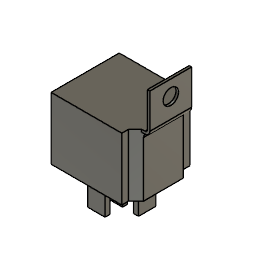
Base (Autodesk Fusion 360 archive; units mm, degrees)
design "Relay BB"
Autodesk Fusion 360 part; units mm, degrees
sketch "Sketch1" plane through (0, 0, 0) normal (0, 0, 1) x (1, 0, 0)
  line L0 (14.2, -13.7) -> (-14.2, -13.7)
  line L1 (-14.2, -13.7) -> (-14.2, 13.7)
  line L2 (-14.2, 13.7) -> (14.2, 13.7)
  line L3 (14.2, 13.7) -> (14.2, -13.7)
  line L4 (14.2, -13.7) -> (-14.2, 13.7) construction
  line L5 (-14.2, -13.7) -> (14.2, 13.7) construction
  dimension "d1" = 28.4
  dimension "d2" = 27.4
  constraint horizontal L0
  constraint perpendicular L0 L1
  constraint parallel L0 L2
  constraint parallel L1 L3
  constraint coincident L4 origin
  constraint coincident L5 origin
  measures "d1" distance of L1.end L2.end
  measures "d2" distance of L0.end L1.end
extrude "Extrude1" add sketch "Sketch1" along normal blind 25
sketch "Sketch2" plane through (14.2, 0, 0) normal (1, 0, 0) x (0, 1, 0)
  line L0 (-13.7, 0) -> (13.7, 0)
  line L1 (13.7, 0) -> (13.7, 25)
  line L2 (13.7, 25) -> (-13.7, 25)
  line L3 (-13.7, 25) -> (-13.7, 0)
  line L4 (0, 25) -> (8.4, 25)
  line L5 (8.4, 25) -> (8.4, 40)
  line L6 (8.4, 40) -> (0, 40)
  line L7 (0, 40) -> (0, 25)
  line L8 (0, 40) -> (-8.4, 40)
  line L9 (-8.4, 40) -> (-8.4, 25)
  line L10 (-8.4, 25) -> (0, 25)
  line L11 (0, 25) -> (0, 40)
  dimension "d5" = 8.4
  dimension "d6" = 15
  dimension "d7" = 8.4
  constraint horizontal L4
  constraint vertical L5
  constraint horizontal L6
  constraint vertical L7
  constraint midpoint L2 L4.start
  constraint horizontal L8
  constraint vertical L9
  constraint horizontal L10
  constraint vertical L11
  constraint coincident L2 L9.end
  measures "d5" distance of L4.start L4.end
  measures "d6" distance of L4.start L6.end
  measures "d7" distance of L6.end L8.end
extrude "Extrude2" add sketch "Sketch2" against normal blind 2 contours L2 L7 L8 L9 L10 L11 | L2 L4 L5 L6 L7 L11
sketch "Sketch3" plane through (14.2, 0, 0) normal (1, 0, 0) x (0, 1, 0)
  line L0 (-13.7, 0) -> (13.7, 0)
  line L1 (13.7, 0) -> (13.7, 25)
  line L2 (13.7, 25) -> (8.4, 25)
  line L3 (-8.4, 25) -> (-13.7, 25)
  line L4 (-13.7, 25) -> (-13.7, 0)
  line L5 (-8.4, 25) -> (8.4, 25)
  line L6 (0, 40) -> (0, 33.9)
  circle A0 centre (0, 33.9) radius 3.1
  line L7 (8.4, 25) -> (8.4, 40)
  line L8 (8.4, 40) -> (-8.4, 40)
  line L9 (-8.4, 40) -> (-8.4, 25)
  dimension "d10" = 6.1
  dimension "d11" = 6.2
  constraint coincident L3.start L5.start
  constraint coincident L2.end L5.end
  constraint coincident L6.end A0.centre
  measures "d10" distance of L6.start L6.end
  measures "d11" diameter of A0
extrude "Extrude3" cut sketch "Sketch3" against normal blind 30 contours A0
sketch "Sketch4" plane through (0, 0, 0) normal (0, 0, 1) x (1, 0, 0)
  line L0 (-3.2, -10) -> (3.8, -10)
  line L1 (3.8, -10) -> (3.8, -8)
  line L2 (3.8, -8) -> (-3.2, -8)
  line L3 (-3.2, -8) -> (-3.2, -10)
  line L4 (-10.2, -3) -> (-8.2, -3)
  line L5 (-8.2, -3) -> (-8.2, 4)
  line L6 (-8.2, 4) -> (-10.2, 4)
  line L7 (-10.2, 4) -> (-10.2, -3)
  line L8 (8.2, -3) -> (10.2, -3)
  line L9 (10.2, -3) -> (10.2, 4)
  line L10 (10.2, 4) -> (8.2, 4)
  line L11 (8.2, 4) -> (8.2, -3)
  line L12 (-3.2, 7.7) -> (3.8, 7.7)
  line L13 (3.8, 7.7) -> (3.8, 9.7)
  line L14 (3.8, 9.7) -> (-3.2, 9.7)
  line L15 (-3.2, 9.7) -> (-3.2, 7.7)
  line L16 (-3.2, -3) -> (3.8, -3)
  line L17 (3.8, -3) -> (3.8, -1)
  line L18 (3.8, -1) -> (-3.2, -1)
  line L19 (-3.2, -1) -> (-3.2, -3)
  line L20 (-14.2, 13.7) -> (14.2, 13.7)
  line L21 (14.2, 13.7) -> (14.2, -13.7)
  line L22 (14.2, -13.7) -> (-14.2, -13.7)
  line L23 (-14.2, -13.7) -> (-14.2, 13.7)
  dimension "d14" = 4
  dimension "d15" = 4
  dimension "d16" = 4
  dimension "d17" = 11
  dimension "d18" = 11
  dimension "d19" = 11
  constraint horizontal L0
  constraint vertical L1
  constraint horizontal L2
  constraint vertical L3
  constraint horizontal L4
  constraint vertical L5
  constraint horizontal L6
  constraint vertical L7
  constraint horizontal L8
  constraint vertical L9
  constraint horizontal L10
  constraint vertical L11
  constraint horizontal L12
  constraint vertical L13
  constraint horizontal L14
  constraint vertical L15
  constraint horizontal L16
  constraint vertical L17
  constraint horizontal L18
  constraint vertical L19
  measures "d14" distance of L9 L21
  measures "d15" distance of L7 L23
  measures "d16" distance of L14 L20
  measures "d17" distance of L15 L23
  measures "d18" distance of L3 L23
  measures "d19" distance of L19 L23
extrude "Extrude4" add sketch "Sketch4" against normal blind 11.3 contours L0 L1 L2 L3 | L4 L5 L6 L7 | L8 L9 L10 L11 | L12 L13 L14 L15 | L16 L17 L18 L19
extrude "Extrude5" add sketch "Sketch3" along normal blind 1 contours L5 L7 L8 L9
sketch "Sketch5" plane through (14.2, 0, 0) normal (1, 0, 0) x (0, 1, 0)
  line L0 (8.4, 25) -> (-8.4, 25)
  line L1 (-8.4, 25) -> (-13.7, 25)
  line L2 (-13.7, 25) -> (-13.7, 0)
  line L3 (-13.7, 0) -> (13.7, 0)
  line L4 (13.7, 0) -> (13.7, 25)
  line L5 (13.7, 25) -> (8.4, 25)
  line L6 (0, 25) -> (11, 25)
  line L7 (11, 25) -> (11, 0)
  line L8 (11, 0) -> (0, 0)
  line L9 (0, 0) -> (0, 25)
  line L10 (0, 25) -> (-11, 25)
  line L11 (-11, 25) -> (-11, 0)
  line L12 (-11, 0) -> (0, 0)
  line L13 (0, 0) -> (0, 25)
  dimension "d26" = 11
  constraint horizontal L6
  constraint vertical L7
  constraint horizontal L8
  constraint vertical L9
  constraint midpoint L0 L6.start
  constraint coincident L3 L7.end
  constraint horizontal L10
  constraint vertical L11
  constraint horizontal L12
  constraint vertical L13
  constraint coincident L3 L11.end
  measures "d26" distance of L6.start L6.end
extrude "Extrude7" add sketch "Sketch5" along normal blind 3 contours L0 L3 L5 L6 L7 L8 L9 L13 | L0 L1 L3 L9 L10 L11 L12 L13
chamfer "Chamfer1" distance 3 angle 45 2 edges at (17.2, -11, 12.5) (17.2, 11, 12.5)
extrude "Extrude8" add 1 faces at (15.2, 0.0772, 26.9362) along direction (1, 0, 0) blind 5
extrude "Extrude9" add 1 faces at (19.2, 2.6669, 25) along direction (0, 0, -1) blind 1
extrude "Extrude10" cut 1 faces at (12.2, -0.0772, 26.9362) along direction (1, 0, 0) blind 7
fillet "Fillet1" radius 2 1 edges at (20.2, 0, 24)
fillet "Fillet2" radius 1 1 edges at (19.2, 0, 25)
fillet "Fillet3" radius 2 1 edges at (17.2, 0, 24)
equation "d5 = ( 16.8 / 2 ) * 1 mm"
equation "d26 = ( 22 / 2 ) * 1 mm"

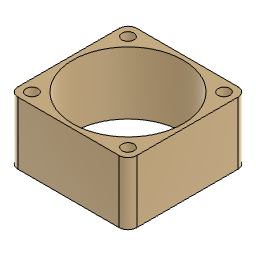
design "noctua_fan_40mm"
Autodesk Fusion 360 part; units mm, degrees
box "BoxPrimitive1" add length 40 width 40 height 21 placed x (0, -1, 0) y (1, 0, 0) z (0, 0, 1) at (40, 0, 0)
fillet "Fillet1" radius 3 4 edges at (40, -40, 10.5) (80, -40, 10.5) (80, 0, 10.5) (40, 0, 10.5)
sketch "Sketch2" plane through (0, 0, 21) normal (0, 0, 1) x (-1, 0, 0)
  arc A0 (-43, 0) -> (-40, 3) centre (-43, 3) ccw
  line L0 (-40, 3) -> (-40, 37)
  arc A1 (-40, 37) -> (-43, 40) centre (-43, 37) ccw
  line L1 (-43, 40) -> (-77, 40)
  arc A2 (-77, 40) -> (-80, 37) centre (-77, 37) ccw
  line L2 (-80, 37) -> (-80, 3)
  arc A3 (-80, 3) -> (-77, 0) centre (-77, 3) ccw
  line L3 (-77, 0) -> (-43, 0)
  circle A4 centre (-76.15, 36.15) radius 2
  circle A5 centre (-76.15, 3.85) radius 2
  circle A6 centre (-43.85, 36.15) radius 2
  circle A7 centre (-43.85, 3.85) radius 2
  line L4 (-40.8787, 0.8787) -> (-79.1213, 39.1213) construction
  line L5 (-40.8787, 39.1213) -> (-79.1213, 0.8787) construction
  circle A8 centre (-60, 20) radius 18.55
  dimension "d8" = 4
  dimension "d9" = 4
  dimension "d10" = 4
  dimension "d11" = 4
  dimension "d12" = 3.85
  dimension "d13" = 3.85
  dimension "d14" = 3.85
  dimension "d15" = 3.85
  dimension "d16" = 3.85
  dimension "d17" = 3.85
  dimension "d18" = 3.85
  dimension "d19" = 3.85
  dimension "d23" = 37.1
  constraint midpoint A0 L4.start
  constraint midpoint A2 L4.end
  constraint midpoint A1 L5.start
  constraint midpoint A3 L5.end
  constraint midpoint L4 A8.centre
  measures "d8" diameter of A4
  measures "d9" diameter of A5
  measures "d10" diameter of A6
  measures "d11" diameter of A7
  measures "d12" distance of L1 A4.centre
  measures "d13" distance of L2 A4.centre
  measures "d14" distance of L3 A5.centre
  measures "d15" distance of L2 A5.centre
  measures "d16" distance of L3 A7.centre
  measures "d17" distance of L0 A7.centre
  measures "d18" distance of L1 A6.centre
  measures "d19" distance of L0 A6.centre
  measures "d23" diameter of A8
extrude "Extrude1" cut sketch "Sketch2" against normal blind 35 contours A4 | A5 | A6 | A7
extrude "Extrude2" cut sketch "Sketch2" against normal blind 35 contours A8
equation "d12 = screw_spacing"
equation "d13 = screw_spacing"
equation "d14 = screw_spacing"
equation "d15 = screw_spacing"
equation "d16 = screw_spacing"
equation "d17 = screw_spacing"
equation "d18 = screw_spacing"
equation "d19 = screw_spacing"
equation "screw_spacing = 3.85 mm"
named bodies: "40mm_fan"
